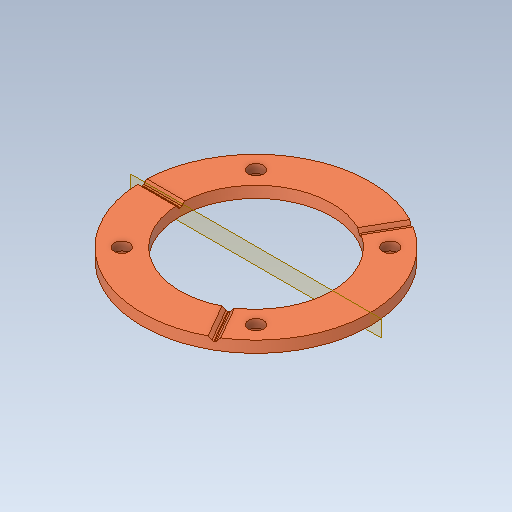
# Autodesk Inventor part: kinematic-mount_base
Saved by Autodesk Inventor 2020.5 (Build 245400000, 400)
## iProperties
Created: 2019-01-08
Part Number: kinematic-mount_base
Material: ABS Plastic
Document SubType Name: Modeling
Designer: Vi Quint Duong
Density: 1.06 g/cm^3
Appearance: Smooth - White
Author: Vi Quint Duong
Autodesk Inventor part; units mm, degrees
ref_plane "YZ Plane" through (0, 0, 0) normal (1, 0, 0) x (0, 1, 0)
ref_plane "XZ Plane" through (0, 0, 0) normal (0, 1, 0) x (-1, 0, 0)
ref_plane "XY Plane" through (0, 0, 0) normal (0, 0, 1) x (1, 0, 0)
sketch "Sketch1" plane through (0, 0, 0) normal (0, 1, 0) x (-1, 0, 0)
  circle A0 centre (0, 0) radius 40
  circle A1 centre (0, 0) radius 60
  dimension "d0" = 80
  dimension "d1" = 120
  constraints: 2 centre point, 2 coincident
  measures "d0" diameter of A0
  measures "d1" diameter of A1
extrude "Extrusion1" add sketch "Sketch1" along normal blind 8
sketch "Sketch2" plane through (0, 8, 0) normal (0, 1, 0) x (1, 0, 0)
  circle A0 centre (0, 0) radius 40 projected
  line L0 (-40, 0) -> (-60, 0)
  circle A1 centre (0, 0) radius 60 projected
  line L1 (20, -34.641) -> (30, -51.9615)
  line L2 (20, 34.641) -> (30, 51.9615)
  circle A2 centre (0, 0) radius 60 projected
  line L3 (-40.0521, 2.5) -> (-59.9479, 2.5)
  line L4 (-59.9479, 2.5) -> (-59.9479, -2.5)
  line L5 (-59.9479, -2.5) -> (-40.0521, -2.5)
  line L6 (-40.0521, -2.5) -> (-40.0521, 2.5)
  line L7 (-40.0521, 2.5) -> (-59.9479, -2.5) construction
  line L8 (-59.9479, 2.5) -> (-40.0521, -2.5) construction
  line L9 (17.861, -35.9361) -> (27.8089, -53.1664)
  line L10 (32.139, -50.6664) -> (22.1911, -33.4361)
  line L11 (22.1911, 33.4361) -> (32.139, 50.6664)
  line L12 (27.8089, 53.1664) -> (17.861, 35.9361)
  point P0 (-50, 0)
  dimension "d6" = 360
  dimension "d8" = 5
  dimension "d11" = 360
  constraints: 26 end point, 3 midpoint, 2 horizontal, 2 horizontal alignment, 2 parallel, 1 perpendicular, 1 point on circle, 31 other
  measures "d8" distance of L4.end L3.end
ref_plane "Work Plane1" through (-60, 8, 0) normal (-1, 0, 0) x (0, -1, 0)
sketch "Sketch3" plane through (-60, 8, 0) normal (-1, 0, 0) x (0, -1, 0)
  line L0 (0.5, 2.2218) -> (0.5, 8.6079) construction
  line L1 (0, 60) -> (0, -60) construction
  line L2 (0, 2.6755) -> (1.9842, 0.8753)
  line L3 (1.9842, 0.8753) -> (1.9842, 0)
  line L4 (1.9842, 0) -> (-4.7604, 0) construction
  line L5 (0.5, 2.2218) -> (2.451, 4.3722) construction
  line L6 (0.5, 2.2218) -> (-1.5158, 0) construction
  circle A0 centre (-1.5158, 0) radius 3 construction
  line L7 (1.4842, 0) -> (1.4842, 1.4538) construction
  line L8 (0, -2.6755) -> (1.9842, -0.8753)
  line L9 (1.9842, -0.8753) -> (1.9842, 0)
  line L10 (0, -2.6755) -> (0, 2.6755)
  point P0 (8, 0)
  point P1 (0, 2.5)
  point P2 (0, 2.5)
  point P3 (0, 2.5)
  point P4 (0, 0)
  dimension "d19" = 0.5
  dimension "d20" = 90
  dimension "d21" = 3
  dimension "d22" = 6
  dimension "d23" = 0.5
  constraints: 20 end point, 4 vertical, 3 point on line, 2 horizontal, 2 symmetric about line, 1 centre point, 1 coincident, 1 perpendicular, 1 tangent
  measures "d19" distance between parallel lines of L1 L0
  measures "d20" angle of L2 L5
  measures "d21" distance of L0.start L6.end
  measures "d22" diameter of A0
  measures "d23" distance between parallel lines of L3 L7
extrude "Extrusion2" cut sketch "Sketch3" against normal up to next
pattern_circular "Circular Pattern1" count 3 over 360 about axis through (0, 0, 0) along (0, 1, 0) of "Extrusion2"
sketch "Sketch4" plane through (0, 8, 0) normal (0, 1, 0) x (1, 0, 0)
  circle A0 centre (0, 0) radius 50
  line L0 (-35.355, 35.355) -> (35.355, 35.355)
  line L1 (35.355, 35.355) -> (35.355, -35.355)
  line L2 (35.355, -35.355) -> (-35.355, -35.355)
  line L3 (-35.355, -35.355) -> (-35.355, 35.355)
  point P0 (-35.355, 0)
  point P1 (0, 35.355)
  dimension "d24" = 100
  dimension "d26" = 70.71
  dimension "d27" = 70.71
  constraints: 8 end point, 5 coincident, 2 midpoint, 2 parallel, 1 centre point, 1 horizontal, 1 horizontal alignment, 1 perpendicular, 1 vertical alignment
  measures "d24" diameter of A0
  measures "d26" distance of L2.end L0.start
  measures "d27" distance of L0.start L0.end
hole "Hole1" at (35.355, 8, 35.355) at (35.355, 8, -35.355) at (-35.355, 8, -35.355) at (-35.355, 8, 35.355) direction (0, -1, 0) diameter 4.4 end through all counterbore diameter 8 counterbore depth 4.5
ref_plane "Work Plane2" through (-50, 8, 0) normal (0, 0, 1) x (0, 1, 0)
thicken "Thicken1" operation add thickness 0.18 both sides no extend neighbours yes toward (0, 0.6719356, -0.7406096) faces at (-46.6513, 6.3467, 1.1754)
thicken "Thicken2" operation add thickness 0.18 both sides no extend neighbours yes toward (0, 0.6719356, 0.7406096) faces at (-46.6513, 6.3467, -1.1754)
thicken "Thicken3" operation add thickness 0.18 both sides no extend neighbours yes toward (-0.6413867, 0.6719356, 0.3703048) faces at (24.3436, 6.3467, 39.8135)
thicken "Thicken4" operation add thickness 0.18 both sides no extend neighbours yes toward (0.6413867, 0.6719356, -0.3703048) faces at (22.3077, 6.3467, 40.9889)
thicken "Thicken5" operation add thickness 0.18 both sides no extend neighbours yes toward (0.6413867, 0.6719356, 0.3703048) faces at (22.3077, 6.3467, -40.9889)
thicken "Thicken6" operation add thickness 0.18 both sides no extend neighbours yes toward (-0.6413867, 0.6719356, -0.3703048) faces at (24.3436, 6.3467, -39.8135)
fillet "Fillet1" radius 1 2 edges at (24.4504, 6.0158, -43.6138) (25.5454, 6.0158, -42.9816)
fillet "Fillet2" radius 1 2 edges at (-49.9958, 6.0158, 0.6322) (-49.9958, 6.0158, -0.6322)
fillet "Fillet3" radius 1 2 edges at (25.5454, 6.0158, 42.9816) (24.4504, 6.0158, 43.6138)
thicken "Thicken7" operation add thickness 2 both sides no extend neighbours yes toward (0, 1, 0) faces at (-41.5413, 0, -27.0926)
body "Solid1"
